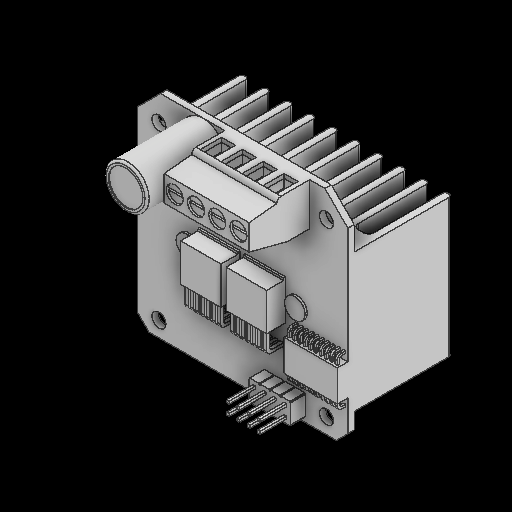
# Autodesk Inventor part: IBT_2
Saved by Autodesk Inventor 2025.2 (Build 292293000, 293)
## iProperties
Created: 2025-11-29
Part Number: IBT_2
Material: Generic
Document SubType Name: Modeling
Designer: valer
Density: 1 g/cm^3
Appearance: Default
Author: valer
Autodesk Inventor part; units mm, degrees
ref_plane "YZ Plane" through (0, 0, 0) normal (1, 0, 0) x (0, 1, 0)
ref_plane "XZ Plane" through (0, 0, 0) normal (0, 1, 0) x (-1, 0, 0)
sketch "Base" plane through (0, 0, 0) normal (0, 0, 1) x (1, 0, 0)
  line L0 (-24.75, -25) -> (24.75, -25)
  line L1 (24.75, -25) -> (24.75, 25)
  line L2 (24.75, 25) -> (-24.75, 25)
  line L3 (-24.75, 25) -> (-24.75, -25)
  line L4 (-24.75, -25) -> (24.75, 25) construction
  line L5 (24.75, -25) -> (-24.75, 25) construction
  point P0 (0, 0)
  dimension "d0" = 50
  dimension "d1" = 49.5
  constraints: 12 end point, 2 midpoint, 2 parallel, 1 horizontal, 1 perpendicular
  measures "d0" distance of L0.end L1.end
  measures "d1" distance of L1.end L2.end
extrude "BaseFeature" add sketch "Base" along normal blind 1.5
chamfer "SmallChamfersFeature" distance 2.7 angle 45 2 edges at (24.75, -25, 0.75) (-24.75, -25, 0.75)
chamfer "LargeChamfersFeature" distance 5.4 angle 45 2 edges at (24.75, 25, 0.75) (-24.75, 25, 0.75)
sketch "MountHoles" plane through (0, 0, 1.5) normal (0, 0, 1) x (1, 0, 0)
  circle A0 centre (19.7, -21.35) radius 1.65
  line L0 (0, -35) -> (0, 35) construction
  line L1 (18.05, -23) -> (21.35, -23) construction
  line L2 (21.35, -23) -> (21.35, -19.7) construction
  line L3 (21.35, -19.7) -> (18.05, -19.7) construction
  line L4 (18.05, -19.7) -> (18.05, -23) construction
  line L5 (18.05, -23) -> (21.35, -19.7) construction
  line L6 (21.35, -23) -> (18.05, -19.7) construction
  line L7 (24.75, -22.3) -> (24.75, 19.6) projected
  line L8 (-22.05, -25) -> (22.05, -25) projected
  circle A1 centre (-19.7, -21.35) radius 1.65
  line L9 (19.7, -21.35) -> (19.7, 18.85) construction
  circle A2 centre (19.7, 18.85) radius 1.65
  line L10 (18.05, 17.2) -> (21.35, 17.2) construction
  line L11 (21.35, 17.2) -> (21.35, 20.5) construction
  line L12 (21.35, 20.5) -> (18.05, 20.5) construction
  line L13 (18.05, 20.5) -> (18.05, 17.2) construction
  line L14 (18.05, 17.2) -> (21.35, 20.5) construction
  line L15 (21.35, 17.2) -> (18.05, 20.5) construction
  line L16 (19.35, 25) -> (-19.35, 25) projected
  circle A3 centre (-19.7, 18.85) radius 1.65
  point P0 (0, 0)
  dimension "d10" = 3.3
  dimension "d11" = 3.4
  dimension "d12" = 2
  dimension "d13" = 4.5
  constraints: 26 end point, 4 centre point, 4 midpoint, 4 parallel, 4 tangent, 2 horizontal, 2 perpendicular, 2 symmetric about line, 1 coincident, 1 equal radius, 1 vertical, 2 other
  measures "d10" diameter of A0
  measures "d11" distance between parallel lines of L7 L2
  measures "d12" distance between parallel lines of L8 L1
  measures "d13" distance between parallel lines of L16 L12
extrude "MountHolesFeature" cut sketch "MountHoles" against normal through all
sketch "Sink" plane through (0, 0, 0) normal (0, 0, -1) x (-1, 0, 0)
  line L0 (-24.75, -22.3) -> (-24.75, 19.6) projected
  line L1 (24.75, 19.6) -> (24.75, -22.3) projected
  line L2 (-24.75, -18.5) -> (24.75, -18.5)
  line L3 (24.75, -18.5) -> (24.75, 14)
  line L4 (24.75, 14) -> (-24.75, 14)
  line L5 (-24.75, 14) -> (-24.75, -18.5)
  line L6 (-19.35, 25) -> (19.35, 25) projected
  line L7 (22.05, -25) -> (-22.05, -25) projected
  point P0 (0, 0)
  point P1 (-24.75, 14)
  point P2 (24.75, -18.5)
  dimension "d16" = 11
  dimension "d17" = 6.5
  constraints: 8 end point, 2 parallel, 2 point on line, 1 horizontal, 1 perpendicular
  measures "d16" distance between parallel lines of L6 L4
  measures "d17" distance between parallel lines of L7 L2
extrude "SinkFeature" add sketch "Sink" along normal blind 23
sketch "SinkRibs" plane through (0, 0, -23) normal (0, 0, -1) x (-1, 0, 0)
  line L0 (-24.75, 14) -> (-24.75, -18.5) projected
  line L1 (-24.75, -18.5) -> (24.75, -18.5) projected
  line L2 (24.75, -18.5) -> (24.75, 14) projected
  line L3 (24.75, 14) -> (-24.75, 14) projected
  line L4 (-24.75, -18.5) -> (24.75, -18.5) projected
  line L5 (-23.15, -18.5) -> (-23.15, 14)
  line L6 (-19.4278, -18.5) -> (-19.4278, 14)
  line L7 (-17.8278, -18.5) -> (-17.8278, 14)
  line L8 (-14.1056, -18.5) -> (-14.1056, 14)
  line L9 (-12.5056, -18.5) -> (-12.5056, 14)
  line L10 (-8.7833, -18.5) -> (-8.7833, 14)
  line L11 (-7.1833, -18.5) -> (-7.1833, 14)
  line L12 (-3.4611, -18.5) -> (-3.4611, 14)
  line L13 (-1.8611, -18.5) -> (-1.8611, 14)
  line L14 (0, -35) -> (0, 35) construction
  line L15 (19.4278, -18.5) -> (19.4278, 14)
  line L16 (17.8278, -18.5) -> (17.8278, 14)
  line L17 (14.1056, -18.5) -> (14.1056, 14)
  line L18 (12.5056, -18.5) -> (12.5056, 14)
  line L19 (8.7833, -18.5) -> (8.7833, 14)
  line L20 (7.1833, -18.5) -> (7.1833, 14)
  line L21 (3.4611, -18.5) -> (3.4611, 14)
  line L22 (1.8611, -18.5) -> (1.8611, 14)
  line L23 (23.15, -18.5) -> (23.15, 14)
  point P0 (0, 0)
  point P1 (8.7833, 14)
  point P2 (7.1833, 14)
  point P3 (3.4611, 14)
  point P4 (1.8611, 14)
  dimension "d20" = 1.6
  dimension "d21" = 1.6
  dimension "d22" = 1.6
  dimension "d23" = 1.6
  dimension "d24" = 3.7222
  dimension "d25" = 3.7222
  dimension "d26" = 3.7222
  dimension "d27" = 1.6
  dimension "d28" = 3.7222
  dimension "d29" = 1.8611
  dimension "d30" = 1.6
  constraints: 36 end point, 16 symmetric about line, 10 vertical, 4 point on line, 18 other
  measures "d20" distance between parallel lines of L0 L5
  measures "d21" distance between parallel lines of L7 L6
  measures "d22" distance between parallel lines of L9 L8
  measures "d23" distance between parallel lines of L11 L10
  measures "d24" distance between parallel lines of L6 L5
  measures "d25" distance between parallel lines of L8 L7
  measures "d26" distance between parallel lines of L10 L9
  measures "d27" distance between parallel lines of L13 L12
  measures "d28" distance between parallel lines of L12 L11
  measures "d29" distance between parallel lines of L14 L13
  measures "d30" distance between parallel lines of L2 L23
ref_plane "SinkBottomPlane" through (0, 0, -5) normal (0, 0, -1) x (-1, 0, 0)
extrude "SinkRibsFeature" cut sketch "SinkRibs" against normal up to surface (18 mm away) contours L3 L6 L1 L5 | L3 L8 L1 L7 | L3 L10 L1 L9 | L3 L12 L1 L11 | L3 L22 L1 L13 | L3 L20 L1 L21 | L3 L18 L1 L19 | L3 L16 L1 L17 | L3 L23 L1 L15
fillet "SinkBottomFilletsFeature" radius 1.25 18 edges at (23.15, -2.25, -5) (19.4278, -2.25, -5) (17.8278, -2.25, -5) (14.1056, -2.25, -5) (8.7833, -2.25, -5) (12.5056, -2.25, -5) (7.1833, -2.25, -5) (3.4611, -2.25, -5) (-1.8611, -2.25, -5) (1.8611, -2.25, -5) (-3.4611, -2.25, -5) (-8.7833, -2.25, -5) (-14.1056, -2.25, -5) (-19.4278, -2.25, -5) (-7.1833, -2.25, -5) (-12.5056, -2.25, -5) (-17.8278, -2.25, -5) (-23.15, -2.25, -5)
fillet "SinkTopFilletsFeature" radius 0.7 20 edges at (24.75, -2.25, -23) (23.15, -2.25, -23) (19.4278, -2.25, -23) (17.8278, -2.25, -23) (14.1056, -2.25, -23) (12.5056, -2.25, -23) (8.7833, -2.25, -23) (7.1833, -2.25, -23) (3.4611, -2.25, -23) (1.8611, -2.25, -23) (-1.8611, -2.25, -23) (-3.4611, -2.25, -23) (-7.1833, -2.25, -23) (-8.7833, -2.25, -23) (-12.5056, -2.25, -23) (-14.1056, -2.25, -23) (-17.8278, -2.25, -23) (-19.4278, -2.25, -23) (-23.15, -2.25, -23) (-24.75, -2.25, -23)
sketch "PinBase" plane through (0, 0, 1.5) normal (0, 0, 1) x (1, 0, 0)
  line L0 (-24.75, -18.5) -> (24.75, -18.5) projected
  line L1 (14.75, -24) -> (5, -24)
  line L2 (5, -24) -> (5, -19)
  line L3 (5, -19) -> (14.75, -19)
  line L4 (14.75, -19) -> (14.75, -24)
  line L5 (24.75, -22.3) -> (24.75, 19.6) projected
  line L6 (-22.05, -25) -> (22.05, -25) projected
  line L7 (12.3125, -19) -> (12.3125, -24) construction
  line L8 (9.875, -19) -> (9.875, -24) construction
  line L9 (7.4375, -19) -> (7.4375, -24) construction
  line L10 (12.1875, -24) -> (12.4375, -24)
  line L11 (12.4375, -24) -> (12.4375, -23.75)
  line L12 (12.4375, -23.75) -> (12.1875, -23.75)
  line L13 (12.1875, -23.75) -> (12.1875, -24)
  line L14 (7.3125, -24) -> (7.3125, -23.75)
  line L15 (7.3125, -23.75) -> (7.5625, -23.75)
  line L16 (7.5625, -23.75) -> (7.5625, -24)
  line L17 (9.75, -24) -> (9.75, -23.75)
  line L18 (9.75, -23.75) -> (10, -23.75)
  line L19 (10, -23.75) -> (10, -24)
  line L20 (5, -21.5) -> (14.75, -21.5) construction
  line L21 (12.4375, -19) -> (12.4375, -19.25)
  line L22 (12.4375, -19.25) -> (12.1875, -19.25)
  line L23 (12.1875, -19.25) -> (12.1875, -19)
  line L24 (7.5625, -19.25) -> (7.5625, -19)
  line L25 (7.3125, -19.25) -> (7.5625, -19.25)
  line L26 (7.3125, -19) -> (7.3125, -19.25)
  line L27 (9.75, -19) -> (9.75, -19.25)
  line L28 (9.75, -19.25) -> (10, -19.25)
  line L29 (10, -19.25) -> (10, -19)
  line L30 (5.125, -19) -> (5.125, -19.25)
  line L31 (5.125, -19.25) -> (5, -19.25)
  line L32 (14.625, -19) -> (14.625, -19.25)
  line L33 (14.625, -19.25) -> (14.75, -19.25)
  line L34 (5.125, -24) -> (5.125, -23.75)
  line L35 (5.125, -23.75) -> (5, -23.75)
  line L36 (14.625, -23.75) -> (14.75, -23.75)
  line L37 (14.625, -24) -> (14.625, -23.75)
  point P0 (0, 0)
  point P1 (12.3125, -23.75)
  point P2 (9.875, -23.75)
  dimension "d36" = 10
  dimension "d37" = 1
  dimension "d38" = 5
  dimension "d39" = 9.75
  dimension "d40" = 2.4375
  dimension "d41" = 2.4375
  dimension "d42" = 2.4375
  dimension "d43" = 2.4375
  dimension "d44" = 0.25
  dimension "d45" = 0.25
  dimension "d46" = 0.125
  constraints: 70 end point, 25 symmetric about line, 11 point on line, 9 perpendicular, 6 midpoint, 4 parallel, 3 equal length, 2 horizontal, 1 vertical
  measures "d36" distance between parallel lines of L5 L4
  measures "d37" distance between parallel lines of L6 L1
  measures "d38" distance of L3.end L1.start
  measures "d39" distance between parallel lines of L4 L2
  measures "d40" distance between parallel lines of L4 L7
  measures "d41" distance between parallel lines of L7 L8
  measures "d42" distance between parallel lines of L9 L8
  measures "d43" distance between parallel lines of L2 L9
  measures "d44" distance of L10.end L11.end
  measures "d45" distance of L11.end L12.end
  measures "d46" distance between parallel lines of L30 L2
extrude "PinBaseFeature" add sketch "PinBase" along normal blind 3.5 contours L1 L11 L12 L13 L19 L18 L17 L16 L15 L14 L34 L35 L2 L31 L30 L3 L26 L25 L24 L27 L28 L29 L23 L22 L21 L32 L33 L4 L36 L37
sketch "Pins" plane through (0, 0, 5) normal (0, 0, 1) x (1, 0, 0)
  line L0 (5, -19.25) -> (5, -23.75) construction
  line L1 (5, -21.5) -> (14.75, -21.5) construction
  line L2 (14.75, -23.75) -> (14.75, -19.25) construction
  line L3 (7.5625, -19.25) -> (7.3125, -19.25) construction
  line L4 (7.4375, -19.25) -> (7.4375, -23.75) construction
  line L5 (7.3125, -23.75) -> (7.5625, -23.75) construction
  line L6 (10, -19.25) -> (9.75, -19.25) construction
  line L7 (9.875, -19.25) -> (9.875, -23.75) construction
  line L8 (9.75, -23.75) -> (10, -23.75) construction
  line L9 (12.4375, -19.25) -> (12.1875, -19.25) construction
  line L10 (12.3125, -19.25) -> (12.3125, -23.75) construction
  line L11 (12.1875, -23.75) -> (12.4375, -23.75) construction
  circle A0 centre (6.2188, -20.2188) radius 1.2188 construction
  line L12 (7.3125, -19) -> (5.125, -19) projected
  line L13 (5.9187, -19.9187) -> (6.5187, -19.9187)
  line L14 (6.5187, -19.9187) -> (6.5187, -20.5187)
  line L15 (6.5187, -20.5187) -> (5.9187, -20.5187)
  line L16 (5.9187, -20.5187) -> (5.9187, -19.9187)
  line L17 (5.9187, -19.9187) -> (6.5187, -20.5187) construction
  line L18 (6.5187, -19.9187) -> (5.9187, -20.5187) construction
  line L19 (8.9488, -19.9187) -> (8.9488, -20.5187)
  line L20 (8.3487, -19.9187) -> (8.9488, -19.9187)
  line L21 (8.9488, -20.5187) -> (8.3487, -20.5187)
  line L22 (8.3487, -20.5187) -> (8.3487, -19.9187)
  line L23 (11.3788, -19.9187) -> (11.3788, -20.5187)
  line L24 (10.7787, -19.9187) -> (11.3788, -19.9187)
  line L25 (11.3788, -20.5187) -> (10.7787, -20.5187)
  line L26 (10.7787, -20.5187) -> (10.7787, -19.9187)
  line L27 (13.8087, -19.9187) -> (13.8087, -20.5187)
  line L28 (13.2088, -19.9187) -> (13.8087, -19.9187)
  line L29 (13.8087, -20.5187) -> (13.2088, -20.5187)
  line L30 (13.2088, -20.5187) -> (13.2088, -19.9187)
  line L31 (6.5187, -22.4187) -> (6.5187, -23.0187)
  line L32 (5.9187, -22.4187) -> (6.5187, -22.4187)
  line L33 (6.5187, -23.0187) -> (5.9187, -23.0187)
  line L34 (5.9187, -23.0187) -> (5.9187, -22.4187)
  line L35 (8.9488, -22.4187) -> (8.9488, -23.0187)
  line L36 (8.3487, -22.4187) -> (8.9488, -22.4187)
  line L37 (8.9488, -23.0187) -> (8.3487, -23.0187)
  line L38 (8.3487, -23.0187) -> (8.3487, -22.4187)
  line L39 (11.3788, -22.4187) -> (11.3788, -23.0187)
  line L40 (10.7787, -22.4187) -> (11.3788, -22.4187)
  line L41 (11.3788, -23.0187) -> (10.7787, -23.0187)
  line L42 (10.7787, -23.0187) -> (10.7787, -22.4187)
  line L43 (13.8087, -22.4187) -> (13.8087, -23.0187)
  line L44 (13.2088, -22.4187) -> (13.8087, -22.4187)
  line L45 (13.8087, -23.0187) -> (13.2088, -23.0187)
  line L46 (13.2088, -23.0187) -> (13.2088, -22.4187)
  point P0 (0, 0)
  dimension "d49" = 0.6
  dimension "d52" = 2.43
  dimension "d55" = 2.5
  constraints: 76 end point, 10 midpoint, 3 tangent, 2 horizontal, 2 parallel, 2 perpendicular, 1 centre point, 1 vertical, 56 other
  measures "d49" distance of L13.start L13.end
  measures "d52" distance of L13.end L19.start
  measures "d55" distance of L13.end L31.start
extrude "PinsFeature" add sketch "Pins" along normal blind 6.2
sketch "Terminal" plane through (0, 0, 1.5) normal (0, 0, 1) x (1, 0, 0)
  line L0 (15.75, 25) -> (-4.25, 25)
  line L1 (-4.25, 25) -> (-4.25, 15)
  line L2 (-4.25, 15) -> (15.75, 15)
  line L3 (15.75, 15) -> (15.75, 25)
  line L4 (24.75, -22.3) -> (24.75, 19.6) projected
  line L5 (19.35, 25) -> (-19.35, 25) projected
  point P0 (0, 0)
  dimension "d60" = 9
  dimension "d61" = 20
  dimension "d62" = 10
  constraints: 8 end point, 2 parallel, 1 collinear, 1 horizontal, 1 perpendicular
  measures "d60" distance between parallel lines of L4 L3
  measures "d61" distance of L0.start L0.end
  measures "d62" distance of L2.end L0.start
extrude "TerminalFeature" add sketch "Terminal" along normal blind 14.25
sketch "TerminalProfile" plane through (15.75, 15, 1.5) normal (1, 0, 0) x (0, 0, -1)
  line L0 (0, 10) -> (0, 0) projected
  line L1 (0, 10) -> (-14.25, 10) projected
  line L2 (-14.25, 0) -> (-14.25, 10) projected
  line L3 (0, 0) -> (-14.25, 0) projected
  line L4 (0, 0) -> (-14.25, 0) projected
  line L5 (-5.25, 0) -> (-14.25, 2.35)
  line L6 (-14.25, 8.35) -> (-7.75, 9)
  line L7 (-7.75, 9) -> (-7.75, 10)
  point P0 (1.5, -15)
  dimension "d65" = 6.5
  dimension "d66" = 9
  dimension "d67" = 6
  dimension "d68" = 1
  dimension "d69" = 2.35
  constraints: 6 end point, 4 point on line, 1 perpendicular
  measures "d65" distance between parallel lines of L2 L7
  measures "d66" distance from line of L2 L5.start
  measures "d67" distance of L6.start L5.end
  measures "d68" distance of L6.end L7.end
  measures "d69" distance of L5.end L2.start
extrude "TerminalProfileFeature" cut sketch "TerminalProfile" against normal through all contours L7 L6 L2 L1 | L3 L2 L5
fillet "TerminalFilletFeature" radius 1 1 edges at (5.75, 25, 9.25)
sketch "TerminalScrews" plane through (0, 0, 15.75) normal (0, 0, 1) x (1, 0, 0)
  line L0 (15.75, 23.35) -> (-4.25, 23.35) projected
  line L1 (15.75, 23.35) -> (-4.25, 23.35) projected
  line L2 (-4.25, 23.35) -> (-4.25, 17.35) projected
  line L3 (-4.25, 17.35) -> (15.75, 17.35) projected
  line L4 (15.75, 17.35) -> (15.75, 23.35) projected
  line L5 (0.75, 23.35) -> (0.75, 17.35) construction
  line L6 (5.75, 23.35) -> (5.75, 17.35) construction
  line L7 (10.75, 23.35) -> (10.75, 17.35) construction
  line L8 (-4.25, 20.35) -> (15.75, 20.35) construction
  line L9 (-4.25, 23.35) -> (-4.25, 17.35) projected
  line L10 (-4.25, 23.35) -> (0.75, 17.35) construction
  line L11 (0.75, 23.35) -> (5.75, 17.35) construction
  line L12 (5.75, 23.35) -> (10.75, 17.35) construction
  line L13 (10.75, 23.35) -> (15.75, 17.35) construction
  circle A0 centre (-1.75, 20.35) radius 2
  circle A1 centre (3.25, 20.35) radius 2
  circle A2 centre (8.25, 20.35) radius 2
  circle A3 centre (13.25, 20.35) radius 2
  point P0 (0, 0)
  dimension "d73" = 5
  dimension "d74" = 5
  dimension "d75" = 5
  dimension "d76" = 5
  dimension "d77" = 4
  constraints: 16 end point, 8 midpoint, 4 centre point, 4 point on line, 3 equal radius, 3 perpendicular
  measures "d73" distance between parallel lines of L5 L2
  measures "d74" distance between parallel lines of L6 L5
  measures "d75" distance between parallel lines of L7 L6
  measures "d76" distance between parallel lines of L4 L7
  measures "d77" diameter of A0
extrude "TerminalScrewsFeature" cut sketch "TerminalScrews" against normal blind 0.5 contours A0 | A1 | A2 | A3
sketch "TerminalScrewHeads" plane through (-1.75, 20.35, 15.25) normal (0, 0, 1) x (1, 0, 0)
  circle A0 centre (0, 0) radius 2 projected
  circle A1 centre (5, 0) radius 2 projected
  circle A2 centre (10, 0) radius 2 projected
  circle A3 centre (15, 0) radius 2 projected
  line L0 (-2, 0) -> (2, 0) construction
  line L1 (17.5, 3.65) -> (-2.5, 3.65) projected
  circle A4 centre (0, 0) radius 2 projected
  line L2 (-1.9843, 0.25) -> (1.9843, 0.25)
  line L3 (-1.9843, -0.25) -> (1.9843, -0.25)
  line L4 (-2.5, 3) -> (-2.5, -3) projected
  line L5 (-1.9843, 0.25) -> (16.9843, 0.25) construction
  circle A5 centre (15, 0) radius 2 projected
  line L6 (3.0157, 0.25) -> (6.9843, 0.25)
  line L7 (8.0157, 0.25) -> (11.9843, 0.25)
  line L8 (13.0157, 0.25) -> (16.9843, 0.25)
  line L9 (3.0157, -0.25) -> (6.9843, -0.25)
  line L10 (8.0157, -0.25) -> (11.9843, -0.25)
  line L11 (13.0157, -0.25) -> (16.9843, -0.25)
  point P0 (1.75, -20.35)
  point P1 (13.0157, -0.25)
  point P2 (16.9843, -0.25)
  point P3 (16.9843, 0.25)
  point P4 (13.0157, 0.25)
  point P5 (1.9843, 0.25)
  point P6 (-1.9843, 0.25)
  dimension "d80" = 0.25
  dimension "d81" = 0.25
  constraints: 20 end point, 18 point on circle, 7 point on line, 4 horizontal, 3 collinear, 1 coincident, 1 midpoint, 1 parallel, 1 perpendicular
  measures "d80" distance between parallel lines of L0 L2
  measures "d81" distance between parallel lines of L3 L0
extrude "TerminalScrewHeadsFeature" cut sketch "TerminalScrewHeads" against normal blind 0.5 contours A0 L3 L2 | A1 L9 L6 | A2 L10 L7 | A3 L11 L8
sketch "TerminalHoles" plane through (-19.35, 25, 0) normal (0, 1, 0) x (1, 0, 0)
  line L0 (35.1, -8.25) -> (15.1, -8.25) construction
  line L1 (35.1, -1.5) -> (35.1, -8.25) construction
  line L2 (38.7, -1.5) -> (35.1, -1.5) construction
  line L3 (38.7, 0) -> (38.7, -1.5) construction
  line L4 (38.7, 0) -> (0, 0) construction
  line L5 (0, -1.5) -> (0, 0) construction
  line L6 (15.1, -1.5) -> (0, -1.5) construction
  line L7 (15.1, -1.5) -> (15.1, -8.25) construction
  line L8 (34.1, -8.25) -> (30.8375, -8.25)
  line L9 (30.8375, -8.25) -> (30.8375, -3.25)
  line L10 (30.8375, -3.25) -> (34.1, -3.25)
  line L11 (34.1, -3.25) -> (34.1, -8.25)
  line L12 (29.1875, -8.25) -> (25.925, -8.25)
  line L13 (25.925, -8.25) -> (25.925, -3.25)
  line L14 (25.925, -3.25) -> (29.1875, -3.25)
  line L15 (29.1875, -3.25) -> (29.1875, -8.25)
  line L16 (24.275, -8.25) -> (21.0125, -8.25)
  line L17 (21.0125, -8.25) -> (21.0125, -3.25)
  line L18 (21.0125, -3.25) -> (24.275, -3.25)
  line L19 (24.275, -3.25) -> (24.275, -8.25)
  line L20 (19.3625, -8.25) -> (16.1, -8.25)
  line L21 (16.1, -8.25) -> (16.1, -3.25)
  line L22 (16.1, -3.25) -> (19.3625, -3.25)
  line L23 (19.3625, -3.25) -> (19.3625, -8.25)
  point P0 (19.35, 0)
  dimension "d84" = 1.65
  dimension "d86" = 1.65
  dimension "d87" = 1.65
  dimension "d88" = 1
  dimension "d89" = 1
  dimension "d90" = 3.2625
  dimension "d91" = 3.2625
  dimension "d92" = 3.2625
  dimension "d93" = 3.2625
  dimension "d95" = 5
  constraints: 32 end point, 8 parallel, 6 point on line, 4 horizontal, 4 perpendicular, 1 collinear
  measures "d84" distance between parallel lines of L23 L17
  measures "d86" distance between parallel lines of L15 L9
  measures "d87" distance between parallel lines of L19 L13
  measures "d88" distance between parallel lines of L1 L11
  measures "d89" distance between parallel lines of L7 L21
  measures "d90" distance of L8.start L8.end
  measures "d91" distance of L12.start L12.end
  measures "d92" distance of L16.start L16.end
  measures "d93" distance of L20.start L20.end
  measures "d95" distance of L10.end L8.start
extrude "TerminalHolesFeature" cut sketch "TerminalHoles" against normal blind 2
chamfer "TerminalChamfersFeature" distance 1 angle 45 16 edges at (11.4875, 23, 5.75) (13.1187, 23, 3.25) (13.1187, 23, 8.25) (14.75, 23, 5.75) (8.2062, 23, 3.25) (9.8375, 23, 5.75) (8.2062, 23, 8.25) (6.575, 23, 5.75) (3.2937, 23, 8.25) (4.925, 23, 5.75) (1.6625, 23, 5.75) (3.2937, 23, 3.25) (0.0125, 23, 5.75) (-1.6188, 23, 8.25) (-1.6188, 23, 3.25) (-3.25, 23, 5.75)
sketch "Capacitor" plane through (0, 0, 1.5) normal (0, 0, 1) x (1, 0, 0)
  circle A0 centre (-9.31, 19.94) radius 5.06
  line L0 (19.35, 25) -> (-19.35, 25) projected
  line L1 (-4.25, 15) -> (-4.25, 25) projected
  point P0 (0, 0)
  dimension "d101" = 10.12
  constraints: 2 tangent, 1 centre point
  measures "d101" diameter of A0
extrude "CapacitorFeature" add sketch "Capacitor" along normal blind 18.25 contours A0
fillet "Fillet4" radius 0.5 1 edges at (-14.37, 19.94, 19.75)
sketch "CapacitorIndent" plane through (-9.31, 19.94, 19.75) normal (0, 0, 1) x (1, 0, 0)
  circle A0 centre (0, 0) radius 4.56 construction
  circle A1 centre (0, 0) radius 4.06
  circle A2 centre (0, 0) radius 5.06 construction
  point P0 (9.31, -19.94)
  dimension "d105" = 1
  constraints: 1 centre point, 1 coincident
  measures "d105" radial gap between concentric circles of A2 A1
extrude "CapacitorIndentFeature" cut sketch "CapacitorIndent" against normal blind 0.25
sketch "SinkScrews" plane through (0, 0, 1.5) normal (0, 0, 1) x (1, 0, 0)
  circle A0 centre (12.75, -2.5) radius 2.44
  line L0 (0, -35) -> (0, 35) construction
  line L1 (24.75, -22.3) -> (24.75, 19.6) projected
  circle A1 centre (-12.75, -2.5) radius 2.44
  line L2 (-22.05, -25) -> (22.05, -25) projected
  point P0 (0, 0)
  dimension "d108" = 4.88
  dimension "d109" = 12
  dimension "d110" = 22.5
  constraints: 2 centre point, 1 symmetric about line, 1 other
  measures "d108" diameter of A0
  measures "d109" distance from line of L1 A0.centre
  measures "d110" distance from line of L2 A0.centre
extrude "SinkScrewsFeature" add sketch "SinkScrews" along normal blind 0.5
sketch "Drivers" plane through (0, 0, 1.5) normal (0, 0, 1) x (1, 0, 0)
  line L0 (0.6111, -18.5) -> (0.6111, 14) construction
  line L1 (0.6111, 1.85) -> (10.1111, 1.85)
  line L2 (10.1111, 1.85) -> (10.1111, -7)
  line L3 (10.1111, -7) -> (0.6111, -7)
  line L4 (0.6111, -7) -> (0.6111, 1.85)
  line L5 (-22.05, -25) -> (22.05, -25) projected
  line L6 (0, -35) -> (0, 35) construction
  line L7 (-0.6111, 1.85) -> (-10.1111, 1.85)
  line L8 (-10.1111, 1.85) -> (-10.1111, -7)
  line L9 (-10.1111, -7) -> (-0.6111, -7)
  line L10 (-0.6111, -7) -> (-0.6111, 1.85)
  point P0 (0, 0)
  dimension "d113" = 9.5
  dimension "d114" = 8.85
  dimension "d115" = 18
  constraints: 16 end point, 4 symmetric about line, 2 parallel, 1 horizontal, 1 perpendicular, 1 point on line
  measures "d113" distance of L1.start L1.end
  measures "d114" distance of L1.end L2.end
  measures "d115" distance between parallel lines of L5 L3
extrude "DriversFeature" add sketch "Drivers" along normal blind 4.5
sketch "DriverLeads" plane through (0, 0, 1.5) normal (0, 0, 1) x (1, 0, 0)
  line L0 (-0.6111, 1.85) -> (-10.1111, 1.85) projected
  line L1 (-10.1111, 1.85) -> (-10.1111, -7) projected
  line L2 (-10.1111, -7) -> (-0.6111, -7) projected
  line L3 (-0.6111, -7) -> (-0.6111, 1.85) projected
  line L4 (0.6111, -7) -> (10.1111, -7) projected
  line L5 (10.1111, -7) -> (10.1111, 1.85) projected
  line L6 (10.1111, 1.85) -> (0.6111, 1.85) projected
  line L7 (0.6111, 1.85) -> (0.6111, -7) projected
  line L8 (-10.1111, 1.85) -> (-0.6111, 1.85)
  line L9 (-0.6111, 1.85) -> (-0.6111, 2.35)
  line L10 (-0.6111, 2.35) -> (-10.1111, 2.35)
  line L11 (-10.1111, 2.35) -> (-10.1111, 1.85)
  line L12 (0.6111, 1.85) -> (10.1111, 1.85) projected
  line L13 (0.6111, 1.85) -> (10.1111, 1.85)
  line L14 (10.1111, 1.85) -> (10.1111, 2.35)
  line L15 (10.1111, 2.35) -> (0.6111, 2.35)
  line L16 (0.6111, 2.35) -> (0.6111, 1.85)
  line L17 (-9.6111, -7) -> (-8.8111, -7)
  line L18 (-8.8111, -7) -> (-8.8111, -12)
  line L19 (-8.8111, -12) -> (-9.6111, -12)
  line L20 (-9.6111, -12) -> (-9.6111, -7)
  line L21 (-8.3411, -12) -> (-8.3411, -7)
  line L22 (-7.5411, -12) -> (-8.3411, -12)
  line L23 (-7.5411, -7) -> (-7.5411, -12)
  line L24 (-7.0711, -12) -> (-7.0711, -7)
  line L25 (-6.2711, -12) -> (-7.0711, -12)
  line L26 (-6.2711, -7) -> (-6.2711, -12)
  line L27 (-5.8011, -12) -> (-5.8011, -7)
  line L28 (-5.0011, -12) -> (-5.8011, -12)
  line L29 (-5.0011, -7) -> (-5.0011, -12)
  line L30 (-4.5311, -12) -> (-4.5311, -7)
  line L31 (-3.7311, -12) -> (-4.5311, -12)
  line L32 (-3.7311, -7) -> (-3.7311, -12)
  line L33 (-3.2611, -12) -> (-3.2611, -7)
  line L34 (-2.4611, -12) -> (-3.2611, -12)
  line L35 (-2.4611, -7) -> (-2.4611, -12)
  line L36 (-1.9911, -12) -> (-1.9911, -7)
  line L37 (-1.1911, -12) -> (-1.9911, -12)
  line L38 (-1.1911, -7) -> (-1.1911, -12)
  line L39 (0, -35) -> (0, 35) construction
  line L40 (8.8111, -7) -> (8.8111, -12)
  line L41 (8.8111, -12) -> (9.6111, -12)
  line L42 (9.6111, -12) -> (9.6111, -7)
  line L43 (8.3411, -12) -> (8.3411, -7)
  line L44 (7.5411, -12) -> (8.3411, -12)
  line L45 (7.5411, -7) -> (7.5411, -12)
  line L46 (7.0711, -12) -> (7.0711, -7)
  line L47 (6.2711, -12) -> (7.0711, -12)
  line L48 (6.2711, -7) -> (6.2711, -12)
  line L49 (5.8011, -12) -> (5.8011, -7)
  line L50 (5.0011, -12) -> (5.8011, -12)
  line L51 (5.0011, -7) -> (5.0011, -12)
  line L52 (4.5311, -12) -> (4.5311, -7)
  line L53 (3.7311, -12) -> (4.5311, -12)
  line L54 (3.7311, -7) -> (3.7311, -12)
  line L55 (3.2611, -12) -> (3.2611, -7)
  line L56 (2.4611, -12) -> (3.2611, -12)
  line L57 (2.4611, -7) -> (2.4611, -12)
  line L58 (1.9911, -12) -> (1.9911, -7)
  line L59 (1.1911, -12) -> (1.9911, -12)
  line L60 (1.1911, -7) -> (1.1911, -12)
  point P0 (0, 0)
  dimension "d118" = 0.5
  dimension "d119" = 5
  dimension "d120" = 0.5
  dimension "d121" = 0.8
  dimension "d124" = 1.27
  constraints: 102 end point, 28 symmetric about line, 7 parallel, 4 horizontal, 3 perpendicular, 1 point on line, 42 other
  measures "d118" distance of L10.end L0.end
  measures "d119" distance of L19.end L17.start
  measures "d120" distance between parallel lines of L20 L1
  measures "d121" distance of L18.end L19.end
  measures "d124" distance of L19.end L21.start
extrude "DriverLeadsBackFeature" add sketch "DriverLeads" along normal blind 0.5 contours L0 L11 L10 L9 | L16 L15 L14 L6
extrude "DriverLeadsFrontFeature" add sketch "DriverLeads" along normal blind 4 contours L38 L37 L36 L2 | L2 L18 L19 L20 | L35 L34 L33 L2 | L2 L23 L22 L21 | L32 L31 L30 L2 | L2 L26 L25 L24 | L29 L28 L27 L2 | L4 L58 L59 L60 | L4 L55 L56 L57 | L42 L41 L40 L4 | L4 L52 L53 L54 | L43 L44 L45 L4 | L4 L49 L50 L51 | L46 L47 L48 L4
fillet "DriverLeadFilletsFeature" radius 1 14 edges at (-9.2111, -12, 5.5) (-7.9411, -12, 5.5) (-6.6711, -12, 5.5) (-5.4011, -12, 5.5) (-4.1311, -12, 5.5) (-2.8611, -12, 5.5) (-1.5911, -12, 5.5) (1.5911, -12, 5.5) (2.8611, -12, 5.5) (4.1311, -12, 5.5) (5.4011, -12, 5.5) (6.6711, -12, 5.5) (7.9411, -12, 5.5) (9.2111, -12, 5.5)
sketch "DriverLeadsProfile" plane through (-9.6111, -12, 1.5) normal (-1, 0, 0) x (0, 0, 1)
  arc A0 (3, 0) -> (4, 1) centre (3, 1) ccw projected
  line L0 (4, 5) -> (4, 1) projected
  line L1 (0, 5) -> (4, 5) projected
  line L2 (0, 0) -> (0, 5) projected
  line L3 (0, 0) -> (3, 0) projected
  line L4 (3.3, 5) -> (3.3, 1.2899)
  line L5 (4, 5) -> (4, 1) projected
  line L6 (0, 0) -> (0, 5) projected
  line L7 (0, 0.7) -> (2.7101, 0.7)
  arc A1 (2.7101, 0.7) -> (3.3, 1.2899) centre (2.7101, 1.2899) ccw
  arc A2 (3, 0) -> (4, 1) centre (3, 1) ccw projected
  line L8 (0, 0) -> (3, 0) projected
  point P0 (-1.5, 12)
  point P1 (0, 0.7)
  dimension "d134" = 0.7
  dimension "d135" = 0.7
  constraints: 4 end point, 3 tangent, 2 parallel, 2 point on circle, 2 point on line, 1 centre point, 1 horizontal
  measures "d134" distance between parallel lines of L3 L7
  measures "d135" distance between parallel lines of L0 L4
extrude "DriverLeadsProfileFeature" cut sketch "DriverLeadsProfile" against normal through all contours L2 L1 L4 A1 L7
sketch "Gate" plane through (0, 0, 1.5) normal (0, 0, 1) x (1, 0, 0)
  line L0 (24.75, -22.3) -> (24.75, 19.6) projected
  line L1 (24.75, -7.64) -> (12.25, -7.64)
  line L2 (12.25, -7.64) -> (12.25, -15)
  line L3 (12.25, -15) -> (24.75, -15)
  line L4 (24.75, -15) -> (24.75, -7.64)
  line L5 (-22.05, -25) -> (22.05, -25) projected
  point P0 (0, 0)
  dimension "d138" = 7.36
  dimension "d139" = 12.5
  dimension "d140" = 10
  constraints: 8 end point, 2 parallel, 1 horizontal, 1 perpendicular, 1 point on line
  measures "d138" distance between parallel lines of L3 L1
  measures "d139" distance between parallel lines of L0 L2
  measures "d140" distance between parallel lines of L3 L5
extrude "GateFeature" add sketch "Gate" along normal blind 2.5
sketch "GateLeads" plane through (0, 0, 1.5) normal (0, 0, 1) x (1, 0, 0)
  line L0 (12.25, -15) -> (24.75, -15) projected
  line L1 (24.75, -15) -> (24.75, -7.64) projected
  line L2 (24.75, -7.64) -> (12.25, -7.64) projected
  line L3 (12.25, -7.64) -> (12.25, -15) projected
  line L4 (12.5056, -18.5) -> (12.5056, 14) construction
  line L5 (12.5056, -7.64) -> (13.0056, -7.64)
  line L6 (13.0056, -7.64) -> (13.0056, -5.64)
  line L7 (13.0056, -5.64) -> (12.5056, -5.64)
  line L8 (12.5056, -5.64) -> (12.5056, -7.64)
  line L9 (12.25, -11.32) -> (24.75, -11.32) construction
  line L10 (13.7556, -5.64) -> (13.7556, -7.64)
  line L11 (14.2556, -5.64) -> (13.7556, -5.64)
  line L12 (14.2556, -7.64) -> (14.2556, -5.64)
  line L13 (15.0056, -5.64) -> (15.0056, -7.64)
  line L14 (15.5056, -5.64) -> (15.0056, -5.64)
  line L15 (15.5056, -7.64) -> (15.5056, -5.64)
  line L16 (16.2556, -5.64) -> (16.2556, -7.64)
  line L17 (16.7556, -5.64) -> (16.2556, -5.64)
  line L18 (16.7556, -7.64) -> (16.7556, -5.64)
  line L19 (17.5056, -5.64) -> (17.5056, -7.64)
  line L20 (18.0056, -5.64) -> (17.5056, -5.64)
  line L21 (18.0056, -7.64) -> (18.0056, -5.64)
  line L22 (18.7556, -5.64) -> (18.7556, -7.64)
  line L23 (19.2556, -5.64) -> (18.7556, -5.64)
  line L24 (19.2556, -7.64) -> (19.2556, -5.64)
  line L25 (20.0056, -5.64) -> (20.0056, -7.64)
  line L26 (20.5056, -5.64) -> (20.0056, -5.64)
  line L27 (20.5056, -7.64) -> (20.5056, -5.64)
  line L28 (21.2556, -5.64) -> (21.2556, -7.64)
  line L29 (21.7556, -5.64) -> (21.2556, -5.64)
  line L30 (21.7556, -7.64) -> (21.7556, -5.64)
  line L31 (22.5056, -5.64) -> (22.5056, -7.64)
  line L32 (23.0056, -5.64) -> (22.5056, -5.64)
  line L33 (23.0056, -7.64) -> (23.0056, -5.64)
  line L34 (23.7556, -5.64) -> (23.7556, -7.64)
  line L35 (24.2556, -5.64) -> (23.7556, -5.64)
  line L36 (24.2556, -7.64) -> (24.2556, -5.64)
  line L37 (13.0056, -15) -> (13.0056, -17)
  line L38 (13.0056, -17) -> (12.5056, -17)
  line L39 (12.5056, -17) -> (12.5056, -15)
  line L40 (13.7556, -17) -> (13.7556, -15)
  line L41 (14.2556, -17) -> (13.7556, -17)
  line L42 (14.2556, -15) -> (14.2556, -17)
  line L43 (15.0056, -17) -> (15.0056, -15)
  line L44 (15.5056, -17) -> (15.0056, -17)
  line L45 (15.5056, -15) -> (15.5056, -17)
  line L46 (16.2556, -17) -> (16.2556, -15)
  line L47 (16.7556, -17) -> (16.2556, -17)
  line L48 (16.7556, -15) -> (16.7556, -17)
  line L49 (17.5056, -17) -> (17.5056, -15)
  line L50 (18.0056, -17) -> (17.5056, -17)
  line L51 (18.0056, -15) -> (18.0056, -17)
  line L52 (18.7556, -17) -> (18.7556, -15)
  line L53 (19.2556, -17) -> (18.7556, -17)
  line L54 (19.2556, -15) -> (19.2556, -17)
  line L55 (20.0056, -17) -> (20.0056, -15)
  line L56 (20.5056, -17) -> (20.0056, -17)
  line L57 (20.5056, -15) -> (20.5056, -17)
  line L58 (21.2556, -17) -> (21.2556, -15)
  line L59 (21.7556, -17) -> (21.2556, -17)
  line L60 (21.7556, -15) -> (21.7556, -17)
  line L61 (22.5056, -17) -> (22.5056, -15)
  line L62 (23.0056, -17) -> (22.5056, -17)
  line L63 (23.0056, -15) -> (23.0056, -17)
  line L64 (23.7556, -17) -> (23.7556, -15)
  line L65 (24.2556, -17) -> (23.7556, -17)
  line L66 (24.2556, -15) -> (24.2556, -17)
  point P0 (0, 0)
  dimension "d143" = 2
  dimension "d144" = 0.5
  dimension "d147" = 1.25
  constraints: 124 end point, 40 symmetric about line, 36 horizontal alignment, 20 parallel, 9 collinear, 2 midpoint, 1 horizontal, 1 perpendicular, 1 point on line, 3 other
  measures "d144" distance of L6.end L7.end
  measures "d147" distance of L7.end L10.start
extrude "GateLeadsFeature" add sketch "GateLeads" along normal blind 2 contours L0 L37 L38 L39 | L8 L7 L6 L2 | L0 L42 L41 L40 | L10 L11 L12 L2 | L0 L45 L44 L43 | L13 L14 L15 L2 | L0 L48 L47 L46 | L16 L17 L18 L2 | L0 L51 L50 L49 | L19 L20 L21 L2 | L0 L54 L53 L52 | L22 L23 L24 L2 | L0 L57 L56 L55 | L25 L26 L27 L2 | L0 L60 L59 L58 | L28 L29 L30 L2 | L0 L63 L62 L61 | L31 L32 L33 L2 | L0 L66 L65 L64 | L34 L35 L36 L2
fillet "GateLeadsFilletsFeature" radius 1 20 edges at (12.7556, -5.64, 3.5) (14.0056, -5.64, 3.5) (15.2556, -5.64, 3.5) (16.5056, -5.64, 3.5) (17.7556, -5.64, 3.5) (19.0056, -5.64, 3.5) (20.2556, -5.64, 3.5) (21.5056, -5.64, 3.5) (22.7556, -5.64, 3.5) (24.0056, -5.64, 3.5) (12.7556, -17, 3.5) (14.0056, -17, 3.5) (15.2556, -17, 3.5) (16.5056, -17, 3.5) (17.7556, -17, 3.5) (19.0056, -17, 3.5) (20.2556, -17, 3.5) (21.5056, -17, 3.5) (22.7556, -17, 3.5) (24.0056, -17, 3.5)
sketch "GateLeadsProfile" plane through (24.2556, -17, 1.5) normal (1, 0, 0) x (0, 0, -1)
  arc A0 (-2, 1) -> (-1, 0) centre (-1, 1) ccw projected
  line L0 (0, 0) -> (-1, 0) projected
  line L1 (0, 2) -> (0, 0) projected
  line L2 (-2, 2) -> (0, 2) projected
  line L3 (-2, 1) -> (-2, 2) projected
  arc A1 (-1.5, 1) -> (-1, 0.5) centre (-1, 1) ccw
  line L4 (-1.5, 1) -> (-1.5, 2)
  line L5 (0, 0.5) -> (-1, 0.5)
  line L6 (-2.5, 2) -> (-2.5, 9.36) projected
  line L7 (0, 2) -> (0, 0) projected
  line L8 (0, 9.36) -> (0, 11.36) projected
  line L9 (0, 2) -> (0, 9.36)
  line L10 (-2.5, 5.68) -> (0, 5.68)
  arc A2 (-1, 10.86) -> (-1.5, 10.36) centre (-1, 10.36) ccw
  line L11 (-1.5, 10.36) -> (-1.5, 9.36)
  line L12 (0, 10.86) -> (-1, 10.86)
  line L13 (0, 9.36) -> (-2, 9.36) projected
  point P0 (1.5, 17)
  point P1 (0, 10.86)
  dimension "d155" = 0.5
  dimension "d156" = 0.5
  constraints: 12 end point, 5 symmetric about line, 4 point on circle, 2 centre point, 2 midpoint, 2 point on line, 1 collinear, 1 tangent, 2 other
  measures "d155" radial gap between concentric circles of A0 A1
  measures "d156" distance between parallel lines of L0 L5
extrude "GateLeadsProfileFeature" cut sketch "GateLeadsProfile" against normal up to surface (11.75 mm away) contours L2 L1 L5 A1 L4 | L13 L11 A2 L12 L8
equation "\"d21\" = d20"
equation "\"d22\" = d20"
equation "\"d23\" = d20"
equation "\"d25\" = d24"
equation "\"d26\" = d24"
equation "\"d27\" = d20"
equation "\"d28\" = d24"
equation "\"d29\" = 0.5 * d24"
equation "\"d30\" = d20"
equation "\"d41\" = d40"
equation "\"d42\" = d40"
equation "\"d43\" = d40"
equation "\"d74\" = d73"
equation "\"d75\" = d73"
equation "\"d76\" = d73"
equation "\"d91\" = d90"
equation "\"d92\" = d90"
equation "\"d93\" = d90"
body "Solid1"
